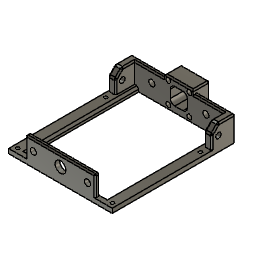
final scissor lift assembly v1 (Autodesk Fusion 360 archive; units mm, degrees)
design "base for scissor lift"
Autodesk Fusion 360 part; units mm, degrees
(part 1 of 2)
sketch "Sketch1" plane through (0, 0, 0) normal (0, 0, 1) x (1, 0, 0)
  line L0 (83.5, 80) -> (-83.5, 80)
  line L1 (-83.5, 80) -> (-83.5, -80)
  line L2 (-83.5, -80) -> (83.5, -80)
  line L3 (83.5, -80) -> (83.5, 80)
  line L4 (83.5, 80) -> (-83.5, -80) construction
  line L5 (-83.5, 80) -> (83.5, -80) construction
  line L6 (-83.5, 80) -> (-86.5, 80)
  line L7 (-86.5, 80) -> (-86.5, -80)
  line L8 (-86.5, -80) -> (-83.5, -80)
  line L9 (-83.5, -80) -> (-83.5, 80)
  line L10 (83.5, 80) -> (86.5, 80)
  line L11 (86.5, 80) -> (86.5, -80)
  line L12 (86.5, -80) -> (83.5, -80)
  line L13 (83.5, -80) -> (83.5, 80)
  dimension "d1" = 167
  dimension "d2" = 160
  dimension "d3" = 3
  dimension "d4" = 160
  dimension "d5" = 3
  dimension "d6" = 160
  constraint horizontal L0
  constraint perpendicular L0 L1
  constraint parallel L0 L2
  constraint parallel L1 L3
  constraint coincident L4 origin
  constraint coincident L5 origin
  constraint horizontal L6
  constraint vertical L7
  constraint horizontal L8
  constraint vertical L9
  constraint horizontal L10
  constraint vertical L11
  constraint horizontal L12
  constraint vertical L13
  measures "d1" distance of L1.end L2.end
  measures "d2" distance of L0.end L1.end
  measures "d3" distance of L0.end L6.end
  measures "d4" distance of L0.end L1.end
  measures "d5" distance of L0.start L10.end
  measures "d6" distance of L0.start L2.end
extrude "Extrude1" add sketch "Sketch1" along normal blind 20 contours L3 L10 L11 L12 L13 | L1 L6 L7 L8 L9 makes body 1 at (86.5, 26.6667, 6.6667) makes body 2 at (-86.5, 26.6667, 6.6667)
sketch "Sketch2" plane through (86.5, 0, 0) normal (1, 0, 0) x (0, 1, 0)
  line L0 (-80, 0) -> (80, 0)
  line L1 (80, 0) -> (80, 20)
  line L2 (80, 20) -> (-80, 20)
  line L3 (-80, 20) -> (-80, 0)
  circle A0 centre (69.9537, 12.5) radius 4
  dimension "d9" = 8
  measures "d9" diameter of A0
extrude "Extrude2" cut sketch "Sketch2" against normal blind 181 contours A0 bodies 1 2
extrude "Extrude4" add sketch "Sketch1" against normal blind 2 bodies 1 2
sketch "Sketch6" plane through (83.5, 0, 0) normal (-1, 0, 0) x (0, -1, 0)
  circle A0 centre (-69.9537, 12.5) radius 4
  line L0 (-80, 0) -> (80, 0)
  line L1 (80, 0) -> (80, 20)
  line L2 (80, 20) -> (-80, 20)
  line L3 (-80, 20) -> (-80, 0)
  line L4 (-80, 20) -> (-60, 20)
  line L5 (-60, 20) -> (-60, 0)
  line L6 (-60, 0) -> (-80, 0)
  line L7 (-80, 0) -> (-80, 20)
  dimension "d31" = 20
  dimension "d32" = 20
  constraint horizontal L4
  constraint vertical L5
  constraint horizontal L6
  constraint vertical L7
  constraint coincident L2.end L3.start
  measures "d31" distance of L2.end L4.end
  measures "d32" distance of L2.end L0.start
extrude "Extrude6" add sketch "Sketch6" along normal blind 18 contours L0 L2 L3 L4 L5 L6 L7 bodies 1
sketch "Sketch7" plane through (-83.5, 0, 0) normal (1, 0, 0) x (0, 1, 0)
  circle A0 centre (69.9537, 12.5) radius 4
  line L0 (-80, 0) -> (80, 0)
  line L1 (80, 0) -> (80, 20)
  line L2 (80, 20) -> (-80, 20)
  line L3 (-80, 20) -> (-80, 0)
  line L4 (80, 20) -> (60, 20)
  line L5 (60, 20) -> (60, 0)
  line L6 (60, 0) -> (80, 0)
  line L7 (80, 0) -> (80, 20)
  dimension "d39" = 20
  dimension "d40" = 20
  constraint horizontal L4
  constraint vertical L5
  constraint horizontal L6
  constraint vertical L7
  constraint coincident L1.end L2.start
  measures "d39" distance of L1.end L4.end
  measures "d40" distance of L1.end L0.end
extrude "Extrude7" add sketch "Sketch7" along normal blind 18 contours L0 L1 L2 L4 L5 L6 L7 bodies 1
sketch "Sketch13" plane through (0, 80, 0) normal (0, 1, 0) x (-1, 0, 0)
  line L0 (-65.5, 20) -> (-86.5, 20)
  line L1 (-86.5, 20) -> (-86.5, -2)
  line L2 (-86.5, -2) -> (86.5, -2)
  line L3 (86.5, -2) -> (86.5, 20)
  line L4 (86.5, 20) -> (65.5, 20)
  line L5 (65.5, 20) -> (65.5, 0)
  line L6 (65.5, 0) -> (-65.5, 0)
  line L7 (-65.5, 0) -> (-65.5, 20)
  line L8 (-86.5, -2) -> (86.5, -2)
  line L9 (86.5, -2) -> (86.5, 20)
  line L10 (86.5, 20) -> (-86.5, 20)
  line L11 (-86.5, 20) -> (-86.5, -2)
  constraint horizontal L8
  constraint vertical L9
  constraint horizontal L10
  constraint vertical L11
  constraint coincident L3.end L4.start
  constraint coincident L1.end L2.start
extrude "Extrude13" add sketch "Sketch13" along normal blind 10 contours L0 L1 L2 L3 L4 L5 L6 L7 L8 L9 L10 L11 bodies 1
extrude "Extrude14" add sketch "Sketch13" along normal blind 2 from surface at 8 contours L5 L6 L7 L10 bodies 1
extrude "Extrude18" cut 1 faces at (-21.8333, -33.3333, 0) along direction (0, 0, -1) blind 2 on bodies 1 bodies 1
sketch "Sketch22" plane through (0, 0, -2) normal (0, 0, -1) x (1, 0, 0)
  line L0 (83.5, 80) -> (83.5, -60)
  line L1 (83.5, -60) -> (65.5, -60)
  line L2 (65.5, -60) -> (65.5, -88)
  line L3 (65.5, -88) -> (-65.5, -88)
  line L4 (-65.5, -88) -> (-65.5, -60)
  line L5 (-65.5, -60) -> (-83.5, -60)
  line L6 (-83.5, -60) -> (-83.5, 80)
  line L7 (-83.5, 80) -> (-86.5, 80)
  line L8 (-86.5, 80) -> (-86.5, -90)
  line L9 (-86.5, -90) -> (86.5, -90)
  line L10 (86.5, -90) -> (86.5, 80)
  line L11 (86.5, 80) -> (83.5, 80)
  line L12 (-86.5, 80) -> (86.5, 80)
  line L13 (86.5, 80) -> (86.5, -90)
  line L14 (86.5, -90) -> (-86.5, -90)
  line L15 (-86.5, -90) -> (-86.5, 80)
  line L16 (86.5, 72.5) -> (103, 72.5)
  line L17 (103, 72.5) -> (103, -82.5)
  line L18 (103, -82.5) -> (86.5, -82.5)
  line L19 (86.5, -82.5) -> (86.5, 72.5)
  line L20 (-86.5, 72.5) -> (-103, 72.5)
  line L21 (-103, 72.5) -> (-103, -82.5)
  line L22 (-103, -82.5) -> (-86.5, -82.5)
  line L23 (-86.5, -82.5) -> (-86.5, 72.5)
  line L24 (-86.5, 80) -> (-91.5, 80)
  line L25 (-91.5, 80) -> (-91.5, 72.5)
  line L26 (-91.5, 72.5) -> (-86.5, 72.5)
  line L27 (-86.5, 72.5) -> (-86.5, 80)
  line L28 (-86.5, -82.5) -> (-91.5, -82.5)
  line L29 (-91.5, -82.5) -> (-91.5, -90)
  line L30 (-91.5, -90) -> (-86.5, -90)
  line L31 (-86.5, -90) -> (-86.5, -82.5)
  line L32 (86.5, 80) -> (91.5, 80)
  line L33 (91.5, 80) -> (91.5, 72.5)
  line L34 (91.5, 72.5) -> (86.5, 72.5)
  line L35 (86.5, 72.5) -> (86.5, 80)
  line L36 (86.5, -90) -> (91.5, -90)
  line L37 (91.5, -90) -> (91.5, -82.5)
  line L38 (91.5, -82.5) -> (86.5, -82.5)
  line L39 (86.5, -82.5) -> (86.5, -90)
  line L40 (-91.5, -90) -> (91.5, -90)
  line L41 (91.5, -90) -> (91.5, -95)
  line L42 (91.5, -95) -> (-91.5, -95)
  line L43 (-91.5, -95) -> (-91.5, -90)
  dimension "d171" = 5
  dimension "d172" = 5
  dimension "d173" = 7.5
  dimension "d174" = 5
  dimension "d175" = 5
  dimension "d176" = 5
  constraint horizontal L12
  constraint vertical L13
  constraint horizontal L14
  constraint vertical L15
  constraint coincident L9.end L10.start
  constraint coincident L7.end L8.start
  constraint horizontal L16
  constraint vertical L17
  constraint horizontal L18
  constraint vertical L19
  constraint coincident L10 L16.start
  constraint horizontal L20
  constraint vertical L21
  constraint horizontal L22
  constraint vertical L23
  constraint coincident L15 L20.start
  constraint horizontal L24
  constraint vertical L25
  constraint horizontal L26
  constraint vertical L27
  constraint horizontal L28
  constraint vertical L29
  constraint horizontal L30
  constraint vertical L31
  constraint horizontal L32
  constraint vertical L33
  constraint horizontal L34
  constraint vertical L35
  constraint horizontal L36
  constraint vertical L37
  constraint horizontal L38
  constraint vertical L39
  constraint horizontal L40
  constraint vertical L41
  constraint horizontal L42
  constraint vertical L43
  measures "d171" distance of L7.end L24.end
  measures "d172" distance of L22.end L28.end
  measures "d173" distance of L28.end L29.end
  measures "d174" distance of L10.end L32.end
  measures "d175" distance of L9.end L36.end
  measures "d176" distance of L29.end L42.end
extrude "Extrude26" add sketch "Sketch22" along normal blind 3 separate body makes body 3
sketch "Sketch23" plane through (0, 0, -2) normal (0, 0, 1) x (-1, 0, 0)
  line L0 (103, 72.5) -> (91.5, 72.5)
  line L1 (91.5, 80) -> (-91.5, 80)
  line L2 (-91.5, 72.5) -> (-103, 72.5)
  line L3 (-103, 72.5) -> (-103, -82.5)
  line L4 (-103, -82.5) -> (-91.5, -82.5)
  line L5 (91.5, -82.5) -> (103, -82.5)
  line L6 (103, -82.5) -> (103, 72.5)
  circle A0 centre (99.32, -80) radius 1.5
  line L7 (91.5, -95) -> (91.5, -82.5)
  line L8 (91.5, 72.5) -> (91.5, 80)
  line L9 (-91.5, 80) -> (-91.5, 72.5)
  line L10 (-91.5, -82.5) -> (-91.5, -95)
  line L11 (-91.5, -95) -> (91.5, -95)
  dimension "d143" = 3
  measures "d143" diameter of A0
extrude "Extrude27" cut sketch "Sketch23" against normal blind 3 contours A0 bodies 3
pattern_linear "R-Pattern5" count 20 spacing 7.8947 along (0, -1, 0) of "Extrude27"
extrude "Extrude29" add 1 faces at (78.5, 79.3333, 20) along direction (0, 0, 1) blind 8 on bodies 1 bodies 1
move_face "OffsetFaces1" offset 5 3 faces at (86.5, -31.3488, 12.8333) (28.8333, 90, 8) (-86.5, -31.3488, 12.8333) on bodies 1
sketch "Sketch30" plane through (0, -80, 0) normal (0, -1, 0) x (1, 0, 0)
  line L0 (-83.5, -2) -> (-83.5, 28)
  line L1 (-83.5, 28) -> (-91.5, 28)
  line L2 (-91.5, 28) -> (-91.5, -2)
  line L3 (-91.5, -2) -> (-83.5, -2)
  line L4 (-91.5, 28) -> (91.5, 28)
  line L5 (91.5, 28) -> (91.5, -2)
  line L6 (91.5, -2) -> (-91.5, -2)
  line L7 (-91.5, -2) -> (-91.5, 28)
  constraint horizontal L4
  constraint vertical L5
  constraint horizontal L6
  constraint vertical L7
  constraint coincident L1.end L2.start
extrude "Extrude36" add sketch "Sketch30" along normal blind 7 bodies 1
sketch "Sketch31" plane through (0, -87, 0) normal (0, -1, 0) x (1, 0, 0)
  line L0 (-91.5, -2) -> (91.5, -2)
  line L1 (91.5, -2) -> (91.5, 28)
  line L2 (91.5, 28) -> (-91.5, 28)
  line L3 (-91.5, 28) -> (-91.5, -2)
  circle A0 centre (0, 12.5) radius 8
  dimension "d193" = 16
  measures "d193" diameter of A0
extrude "Extrude37" cut sketch "Sketch31" against normal blind 7 contours A0 bodies 1
sketch "Sketch32" plane through (0, -87, 0) normal (0, -1, 0) x (1, 0, 0)
  circle A0 centre (0, 12.5) radius 8
  line L0 (-91.5, -2) -> (91.5, -2)
  line L1 (91.5, -2) -> (91.5, 28)
  line L2 (91.5, 28) -> (-91.5, 28)
  line L3 (-91.5, 28) -> (-91.5, -2)
  circle A1 centre (-40, 12.5) radius 4.5
  circle A2 centre (40, 12.5) radius 4.5
  line L4 (40, 12.5) -> (0, 12.5)
  line L5 (0, 12.5) -> (-40, 12.5)
  dimension "d206" = 9
  dimension "d207" = 9
  dimension "d214" = 40
  dimension "d215" = 40
  constraint coincident A2.centre L4.start
  constraint parallel L2 L4
  constraint parallel L4 L5
  measures "d206" diameter of A1
  measures "d207" diameter of A2
  measures "d214" distance of A2.centre A0.centre
  measures "d215" distance of A0.centre A1.centre
extrude "Extrude38" cut sketch "Sketch32" against normal blind 182 contours A1 | A2 bodies 1
sketch "Sketch35" plane through (0, 0, -2) normal (0, 0, -1) x (1, 0, 0)
  line L0 (-91.5, 87) -> (-91.5, -95)
  line L1 (-91.5, -95) -> (91.5, -95)
  line L2 (91.5, -95) -> (91.5, 87)
  line L3 (91.5, 87) -> (-91.5, 87)
  line L4 (-83.5, 80) -> (83.5, 80)
  line L5 (83.5, 80) -> (83.5, -60)
  line L6 (83.5, -60) -> (65.5, -60)
  line L7 (65.5, -60) -> (65.5, -88)
  line L8 (65.5, -88) -> (-65.5, -88)
  line L9 (-65.5, -88) -> (-65.5, -60)
  line L10 (-65.5, -60) -> (-83.5, -60)
  line L11 (-83.5, -60) -> (-83.5, 80)
  line L12 (-91.5, 87) -> (91.5, 87)
  line L13 (91.5, 87) -> (91.5, -95)
  line L14 (91.5, -95) -> (-91.5, -95)
  line L15 (-91.5, -95) -> (-91.5, 87)
  line L16 (-49.9161, -98) -> (-91.5, -98)
  line L17 (-91.5, -98) -> (-91.5, -95)
  line L18 (-91.5, -95) -> (-49.9161, -95)
  line L19 (-49.9161, -95) -> (-49.9161, -98)
  constraint horizontal L12
  constraint vertical L13
  constraint horizontal L14
  constraint vertical L15
  constraint coincident L1.end L2.start
  constraint coincident L0.start L3.end
  constraint horizontal L16
  constraint vertical L17
  constraint horizontal L18
  constraint vertical L19
  constraint coincident L0.end L1.start
extrude "Extrude41" add sketch "Sketch35" along normal blind 6.65 contours L0 L1 L2 L3 L12 L13 L14 L15 L18 | L4 L5 L6 L7 L8 L9 L10 L11 bodies 1
sketch "Sketch36" plane through (0, 0, -2) normal (0, 0, 1) x (-1, 0, 0)
  line L0 (65.5, -60) -> (83.5, -60)
  line L1 (83.5, -60) -> (83.5, 80)
  line L2 (83.5, 80) -> (-83.5, 80)
  line L3 (-83.5, 80) -> (-83.5, -60)
  line L4 (-83.5, -60) -> (-65.5, -60)
  line L5 (-65.5, -60) -> (-65.5, -88)
  line L6 (-65.5, -88) -> (65.5, -88)
  line L7 (65.5, -88) -> (65.5, -60)
sketch "Sketch37" plane through (0, 0, -2) normal (0, 0, 1) x (-1, 0, 0)
  line L0 (65.5, -60) -> (83.5, -60)
  line L1 (83.5, -60) -> (83.5, 80)
  line L2 (83.5, 80) -> (-83.5, 80)
  line L3 (-83.5, 80) -> (-83.5, -60)
  line L4 (-83.5, -60) -> (-65.5, -60)
  line L5 (-65.5, -60) -> (-65.5, -88)
  line L6 (-65.5, -88) -> (65.5, -88)
  line L7 (65.5, -88) -> (65.5, -60)
  line L8 (-83.5, 80) -> (-59.3, 80)
  line L9 (-59.3, 80) -> (-59.3, -88)
  line L10 (-59.3, -88) -> (-83.5, -88)
  line L11 (-83.5, -88) -> (-83.5, 80)
  line L12 (83.5, 80) -> (59.3, 80)
  line L13 (59.3, 80) -> (59.3, -88)
  line L14 (59.3, -88) -> (83.5, -88)
  line L15 (83.5, -88) -> (83.5, 80)
  dimension "d264" = 24.2
  dimension "d265" = 24.2
  dimension "d266" = 168
  dimension "d267" = 168
  constraint horizontal L8
  constraint vertical L9
  constraint horizontal L10
  constraint vertical L11
  constraint coincident L6 L9.end
  constraint coincident L2.end L3.start
  constraint horizontal L12
  constraint vertical L13
  constraint horizontal L14
  constraint vertical L15
  constraint coincident L1.end L2.start
  measures "d264" distance of L2.end L8.end
  measures "d265" distance of L1.end L12.end
  measures "d266" distance of L8.end L9.end
  measures "d267" distance of L12.end L13.end
extrude "Extrude43" cut sketch "Sketch37" against normal blind 6.65 contours L2 L6 L9 L13 bodies 1
chamfer "Chamfer2" distance 3 angle 45 2 edges at (-59.3, 4, -2) (59.3, 4, -2) on bodies 1
sketch "Sketch39" plane through (0, 95, 0) normal (0, 1, 0) x (-1, 0, 0)
  circle A0 centre (-31.5, 2.5) radius 1.4
  circle A1 centre (31.5, 12.5) radius 1.4
  circle A2 centre (0, 22.5) radius 1.4
  circle A3 centre (-31.5, 12.5) radius 1.4
  circle A4 centre (0, 2.5) radius 1.4
  circle A5 centre (31.5, 22.5) radius 1.4
  circle A6 centre (31.5, 2.5) radius 1.4
  circle A7 centre (-31.5, 22.5) radius 1.4
  circle A8 centre (0, 12.5) radius 4.5
  circle A9 centre (-40, 12.5) radius 4.5
  circle A10 centre (40, 12.5) radius 4.5
  line L0 (-91.5, 28) -> (-91.5, -8.65)
  line L1 (-91.5, -8.65) -> (91.5, -8.65)
  line L2 (91.5, -8.65) -> (91.5, 28)
  line L3 (91.5, 28) -> (-91.5, 28)
  line L4 (-21.15, 33.65) -> (21.15, 33.65)
  line L5 (21.15, 33.65) -> (21.15, -8.65)
  line L6 (21.15, -8.65) -> (-21.15, -8.65)
  line L7 (-21.15, -8.65) -> (-21.15, 33.65)
  circle A11 centre (15.5, 28) radius 1.6
  circle A12 centre (-15.5, 28) radius 1.6
  circle A13 centre (15.5, -3) radius 1.6
  circle A14 centre (-15.5, -3) radius 1.6
  circle A15 centre (-40, 12.5) radius 4.5
  circle A16 centre (40, 12.5) radius 4.5
  circle A17 centre (0, 12.5) radius 8
  line L8 (83.5, -2) -> (83.5, 28)
  line L9 (83.5, 28) -> (-83.5, 28)
  line L10 (-83.5, 28) -> (-83.5, -2)
  line L11 (-83.5, -2) -> (-62.3, -2)
  line L12 (-62.3, -2) -> (-59.3, -5)
  line L13 (-59.3, -5) -> (-59.3, -8.65)
  line L14 (-59.3, -8.65) -> (59.3, -8.65)
  line L15 (59.3, -8.65) -> (59.3, -5)
  line L16 (59.3, -5) -> (62.3, -2)
  line L17 (62.3, -2) -> (83.5, -2)
  circle A18 centre (-40, 12.5) radius 4.5
  circle A19 centre (40, 12.5) radius 4.5
  line L18 (-91.5, 28) -> (-91.5, -8.65)
  line L19 (-91.5, -8.65) -> (91.5, -8.65)
  line L20 (91.5, -8.65) -> (91.5, 28)
  line L21 (91.5, 28) -> (-91.5, 28)
  point P0 (0, 12.5)
  dimension "d287" = 42.3
  dimension "d288" = 3.2
  dimension "d289" = 3.2
  dimension "d290" = 3.2
  dimension "d291" = 3.2
  constraint horizontal L4
  constraint perpendicular L4 L5
  constraint parallel L4 L6
  constraint parallel L5 L7
  constraint coincident P0 A8.centre
  constraint coincident L3 A11.centre
  constraint coincident L3 A12.centre
  measures "d287" distance of L5.end L6.end
  measures "d288" diameter of A11
  measures "d289" diameter of A12
  measures "d290" diameter of A13
  measures "d291" diameter of A14
extrude "Extrude45" add sketch "Sketch39" against normal blind 7 contours L3 L4 L5 L7 A11 A12 L9 L21 bodies 1
extrude "Extrude46" cut sketch "Sketch39" against normal blind 7 contours L3 A12 L9 L21 | L3 A11 L9 L21 | A13 | A14 picked at (-15.6948, 27.5035) picked at (15.3052, 27.3446) bodies 1
extrude "Extrude48" cut 1 faces at (-83.5, 13.3333, 8) along direction (1, 0, 0) blind -30 and the other way blind -220 on bodies 1 bodies 1
sketch "Sketch41" plane through (0, 95, 0) normal (0, -1, 0) x (1, 0, 0)
  circle A0 centre (40, 12.5) radius 4.5
  circle A1 centre (-40, 12.5) radius 4.5
  line L0 (21.15, 28) -> (21.15, 33.65)
  line L1 (21.15, 33.65) -> (-21.15, 33.65)
  line L2 (-21.15, 33.65) -> (-21.15, 28)
  line L3 (-21.15, 28) -> (-65.5, 28)
  line L4 (-59.3, -8.65) -> (59.3, -8.65)
  line L5 (65.5, 28) -> (21.15, 28)
  line L6 (-21.15, 33.65) -> (21.15, 33.65)
  line L7 (21.15, 33.65) -> (21.15, -8.65)
  line L8 (21.15, -8.65) -> (-21.15, -8.65)
  line L9 (-21.15, -8.65) -> (-21.15, 33.65)
  line L10 (-21.15, 33.65) -> (21.15, -8.65) construction
  line L11 (21.15, 33.65) -> (-21.15, -8.65) construction
  line L12 (-12.5, 25) -> (12.5, 25)
  line L13 (12.5, 25) -> (12.5, 0)
  line L14 (12.5, 0) -> (-12.5, 0)
  line L15 (-12.5, 0) -> (-12.5, 25)
  line L16 (-12.5, 25) -> (12.5, 0) construction
  line L17 (12.5, 25) -> (-12.5, 0) construction
  circle A2 centre (0, 12.5) radius 4.5
  line L18 (-65.5, 28) -> (-65.5, -2)
  line L19 (-65.5, -2) -> (-62.3, -2)
  line L20 (-62.3, -2) -> (-59.3, -5)
  line L21 (-59.3, -5) -> (-59.3, -8.65)
  line L22 (59.3, -8.65) -> (59.3, -5)
  line L23 (59.3, -5) -> (62.3, -2)
  line L24 (62.3, -2) -> (65.5, -2)
  line L25 (65.5, -2) -> (65.5, 28)
  circle A3 centre (15.5, 28) radius 1.6
  circle A4 centre (-15.5, 28) radius 1.6
  circle A5 centre (15.5, -3) radius 1.6
  circle A6 centre (-15.5, -3) radius 1.6
  line L26 (21.15, 28) -> (91.5, 28)
  line L27 (91.5, 28) -> (91.5, -8.65)
  line L28 (91.5, -8.65) -> (-91.5, -8.65)
  line L29 (-91.5, -8.65) -> (-91.5, 28)
  line L30 (-91.5, 28) -> (-21.15, 28)
  line L31 (-21.15, 28) -> (-21.15, 33.65)
  line L32 (-21.15, 33.65) -> (21.15, 33.65)
  line L33 (21.15, 33.65) -> (21.15, 28)
  circle A7 centre (40, 12.5) radius 4.5
  circle A8 centre (-40, 12.5) radius 4.5
  point P0 (0, 12.5)
  point P1 (0, 12.5)
  dimension "d308" = 25
  dimension "d309" = 25
  constraint horizontal L6
  constraint perpendicular L6 L7
  constraint parallel L6 L8
  constraint parallel L7 L9
  constraint coincident L10 P1
  constraint coincident L11 P1
  constraint coincident L1.end L2.start
  constraint horizontal L12
  constraint perpendicular L12 L13
  constraint parallel L12 L14
  constraint parallel L13 L15
  constraint coincident L16 P1
  constraint coincident L17 P1
  measures "d308" distance of L13.end L14.end
  measures "d309" distance of L12.end L13.end
extrude "Extrude49" add sketch "Sketch41" against normal blind 17.7 contours L0 L1 L2 L4 L6 L7 L8 L9 L28 L31 L32 L33 bodies 1
sketch "Sketch42" plane through (0, -80, 0) normal (0, 1, 0) x (-1, 0, 0)
  line L0 (91.5, 28) -> (-91.5, 28)
  line L1 (-91.5, 28) -> (-91.5, -2)
  line L2 (-91.5, -2) -> (-62.3, -2)
  line L3 (-62.3, -2) -> (-59.3, -5)
  line L4 (-59.3, -5) -> (-59.3, -8.65)
  line L5 (-59.3, -8.65) -> (59.3, -8.65)
  line L6 (59.3, -8.65) -> (59.3, -5)
  line L7 (59.3, -5) -> (62.3, -2)
  line L8 (62.3, -2) -> (91.5, -2)
  line L9 (91.5, -2) -> (91.5, 28)
  circle A0 centre (0, 12.5) radius 8
  circle A1 centre (40, 12.5) radius 4.5
  circle A2 centre (-40, 12.5) radius 4.5
  line L10 (-91.5, 28) -> (-51.5, 28)
  line L11 (-51.5, 28) -> (-51.5, -2)
  line L12 (-51.5, -2) -> (-91.5, -2)
  line L13 (-91.5, -2) -> (-91.5, 28)
  line L14 (91.5, 28) -> (51.5, 28)
  line L15 (51.5, 28) -> (51.5, -2)
  line L16 (51.5, -2) -> (91.5, -2)
  line L17 (91.5, -2) -> (91.5, 28)
  dimension "d312" = 40
  dimension "d313" = 40
  constraint horizontal L10
  constraint vertical L11
  constraint horizontal L12
  constraint vertical L13
  constraint coincident L0.end L1.start
  constraint horizontal L14
  constraint vertical L15
  constraint horizontal L16
  constraint vertical L17
  constraint coincident L0.start L9.end
  measures "d312" distance of L0.end L10.end
  measures "d313" distance of L0.start L14.end
extrude "Extrude50" cut sketch "Sketch42" against normal blind 35 contours L0 L8 L9 L14 L15 L16 L17 | L0 L1 L2 L10 L11 L12 L13 bodies 1
extrude "Extrude51" cut 2 faces at (91.5, 22.6667, -6.4333) (91.5, 87.9846, 12.8333) along direction (-1, 0, 0) blind 15 on bodies 1 bodies 1
extrude "Extrude52" cut 1 faces at (-91.5, 87.9697, 10.4179) along direction (1, 0, 0) blind 15 on bodies 1 bodies 1
chamfer "Chamfer3" distance 10 angle 45 2 edges at (-71, 60, 28) (71, 60, 28) on bodies 1
chamfer "Chamfer4" distance 2 angle 45 41 edges at (-65.5, 60, 8) (-76.5, 60, 8) (-76.5, 65, 23) (-71, 60, 18) (-65.5, 65, 23) (-71, 70, 28) (-76.5, 82.5, 28) (-65.5, 79, 28) (-48.825, 95, 28) (48.825, 95, 28) (43.325, 88, 28) (-43.325, 88, 28) (76.5, 82.5, 28) (65.5, 79, 28) (65.5, 65, 23) (71, 70, 28) (76.5, 65, 23) (71, 60, 18) (65.5, 60, 8) (76.5, 60, 8) (76.5, 95, 9.675) (-76.5, 95, 9.675) (56.325, 95, 28) (0, -80, 28) (43.325, 88, 28) (0, -87, 28) (51.5, -83.5, 28) (-43.325, 88, 28) (0, -87, 28) (-51.5, -83.5, 28) (-56.325, 95, 28) (0, -80, 28) (51.5, -87, 13) (51.5, -80, 13) (-51.5, -80, 13) (-51.5, -87, 13) (-21.15, 112.7, 12.5) (21.15, 112.7, 12.5) (-21.15, 103.85, -8.65) (21.15, 103.85, -8.65) (0, 112.7, -8.65) 1 faces at (-7.05, 96.2333, 33.65) on bodies 1
sketch "Sketch44" plane through (0, 0, -2) normal (0, 0, 1) x (-1, 0, 0)
  line L0 (76.5, -62) -> (76.5, 87)
  line L1 (76.5, 87) -> (49.5, 87)
  line L2 (49.5, 87) -> (51.5, 85)
  line L3 (51.5, 85) -> (51.5, 82)
  line L4 (51.5, 82) -> (49.5, 80)
  line L5 (49.5, 80) -> (62.3, 80)
  line L6 (62.3, 80) -> (62.3, -88)
  line L7 (62.3, -88) -> (65.5, -88)
  line L8 (65.5, -88) -> (65.5, -62)
  line L9 (65.5, -62) -> (67.5, -60)
  line L10 (67.5, -60) -> (74.5, -60)
  line L11 (74.5, -60) -> (76.5, -62)
  circle A0 centre (-70, 80) radius 2.5
  dimension "d322" = 5
  measures "d322" diameter of A0
extrude "Extrude53" cut sketch "Sketch44" against normal blind 10 contours A0 bodies 1
pattern_linear "R-Pattern7" count 2 spacing 130 along (0, 1, 0) count 2 spacing 140 along (-1, 0, 0) of "Extrude53"
sketch "Sketch45" plane through (0, 88, 0) normal (0, -1, 0) x (1, 0, 0)
  line L0 (21.15, 31.65) -> (-21.15, 31.65)
  line L1 (-21.15, 31.65) -> (-21.15, 26)
  line L2 (-21.15, 26) -> (-65.5, 26)
  line L3 (-65.5, 26) -> (-65.5, -2)
  line L4 (-65.5, -2) -> (-62.3, -2)
  line L5 (-62.3, -2) -> (-59.3, -5)
  line L6 (-59.3, -5) -> (-59.3, -8.65)
  line L7 (-59.3, -8.65) -> (59.3, -8.65)
  line L8 (59.3, -8.65) -> (59.3, -5)
  line L9 (59.3, -5) -> (62.3, -2)
  line L10 (62.3, -2) -> (65.5, -2)
  line L11 (65.5, -2) -> (65.5, 26)
  line L12 (65.5, 26) -> (21.15, 26)
  line L13 (21.15, 26) -> (21.15, 31.65)
  circle A0 centre (15.5, -3) radius 1.6
  circle A1 centre (-15.5, -3) radius 1.6
  circle A2 centre (15.5, 28) radius 1.6
  circle A3 centre (-15.5, 28) radius 1.6
  circle A4 centre (40, 12.5) radius 4.5
  circle A5 centre (-40, 12.5) radius 4.5
  circle A6 centre (-15.5, 28) radius 3.5
  circle A7 centre (-15.5, -3) radius 3.5
  circle A8 centre (15.5, -3) radius 3.5
  circle A9 centre (15.5, 28) radius 3.5
  dimension "d329" = 7
  dimension "d330" = 7
  dimension "d331" = 7
  dimension "d332" = 7
  constraint concentric A3 A6
  constraint concentric A1 A7
  constraint concentric A0 A8
  constraint concentric A2 A9
  measures "d329" diameter of A6
  measures "d330" diameter of A7
  measures "d331" diameter of A8
  measures "d332" diameter of A9
extrude "Extrude54" cut sketch "Sketch45" against normal blind 15.7 contours A6 | A7 | A8 | A9 bodies 1
extrude "Extrude55" cut 1 faces at (-4.1667, 95, 8.3333) along direction (0, -1, 0) blind 7 on bodies 1 bodies 1
fillet "Fillet2" radius 6.5 4 edges at (-12.5, 100.35, 25) (-12.5, 100.35, 0) (12.5, 100.35, 25) (12.5, 100.35, 0) on bodies 1
sketch "Sketch46" plane through (0, 0, 0) normal (0, 0, 1) x (1, 0, 0)
  line L0 (-21, 88) -> (-21, 113)
  line L1 (-21, 113) -> (-80, 113)
  line L2 (-80, 113) -> (-80, -100)
  line L3 (-80, -100) -> (100, -100)
  line L4 (100, -100) -> (100, 100)
  line L5 (100, 100) -> (21.9148, 113)
  line L6 (21.9148, 113) -> (21.9148, 88.2807)
  line L7 (21.9148, 88.2807) -> (-21, 88)
  constraint vertical L0
  constraint perpendicular L0 L1
  constraint perpendicular L1 L2
  constraint perpendicular L2 L3
  constraint perpendicular L3 L4
  constraint parallel L4 L6
sketch "Sketch47" plane through (0, 95, 0) normal (0, 1, 0) x (-1, 0, 0)
  line L0 (-74.5, 26) -> (-74.5, -8.65)
  line L1 (-74.5, -8.65) -> (-19.15, -8.65)
  line L2 (-19.15, -8.65) -> (-21.15, -6.65)
  line L3 (-21.15, -6.65) -> (-21.15, 26)
  line L4 (-21.15, 26) -> (-74.5, 26)
  circle A0 centre (-40, 12.5) radius 4.5
  circle A1 centre (-40, 12.5) radius 6
  circle A2 centre (40, 12.5) radius 6
  dimension "d343" = 12
  dimension "d344" = 12
  constraint concentric A0 A1
  measures "d343" diameter of A1
  measures "d344" diameter of A2
extrude "Extrude58" add sketch "Sketch47" along normal blind 2 contours A0 | A1 | A2 bodies 1
fillet "Fillet3" radius 2 2 edges at (-34.406, 95, 14.6697) (45.594, 95, 14.6697) on bodies 1
hidden bodies 3
equation "d264 = 12.100 * 2 mm"
equation "d333 = -20.00 mm + 4.3 mm"

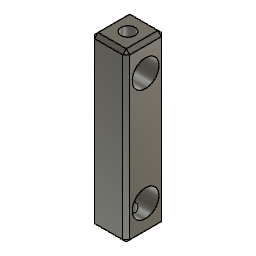
design "small slider"
Autodesk Fusion 360 part; units mm, degrees
sketch "Sketch1" plane through (0, 0, 0) normal (0, 0, 1) x (1, 0, 0)
  line L0 (10, -11) -> (-10, -11)
  line L1 (-10, -11) -> (-10, 11)
  line L2 (-10, 11) -> (10, 11)
  line L3 (10, 11) -> (10, -11)
  line L4 (10, -11) -> (-10, 11) construction
  line L5 (-10, -11) -> (10, 11) construction
  circle A0 centre (0, 0) radius 4
  dimension "d1" = 20
  dimension "d2" = 22
  dimension "d75" = 8
  constraint horizontal L0
  constraint perpendicular L0 L1
  constraint parallel L0 L2
  constraint parallel L1 L3
  measures "d1" distance of L1.end L2.end
  measures "d2" distance of L0.end L1.end
  measures "d75" diameter of A0
extrude "Extrude1" add sketch "Sketch1" along normal blind 95 contours L0 L1 L2 L3 | A0
sketch "Sketch3" plane through (0, 0, 95) normal (0, 0, 1) x (-1, 0, 0)
  line L0 (-10, -11) -> (10, -11)
  line L1 (10, -11) -> (10, 11)
  line L2 (10, 11) -> (-10, 11)
  line L3 (-10, 11) -> (-10, -11)
  circle A0 centre (0, 0) radius 4
  dimension "d21" = 8
  measures "d21" diameter of A0
extrude "Extrude5" cut sketch "Sketch3" against normal blind 10 contours A0
extrude "Extrude6" cut sketch "Sketch1" along normal blind 10 contours A0
sketch "Sketch5" plane through (10, 0, 0) normal (1, 0, 0) x (0, 1, 0)
  line L0 (-11, 0) -> (11, 0)
  line L1 (11, 0) -> (11, 95)
  line L2 (-11, 95) -> (-11, 0)
  circle A0 centre (0, 15.5) radius 7.6
  circle A1 centre (0, 79.5) radius 7.6
  line L3 (11, 95) -> (-11, 95)
  line L4 (0, 95) -> (0, 79.5)
  dimension "d41" = 15.2
  dimension "d43" = 15.2
  dimension "d97" = 15.5
  constraint midpoint L3 L4.start
  constraint perpendicular L3 L4
  measures "d41" diameter of A0
  measures "d43" diameter of A1
  measures "d97" distance of L4.start A1.centre
extrude "Extrude8" cut sketch "Sketch5" against normal blind 20 contours A0 | A1
sketch "Sketch6" plane through (-10, 0, 0) normal (-1, 0, 0) x (0, -1, 0)
  circle A0 centre (0, 15.5) radius 7.6
  line L0 (-11, 0) -> (11, 0)
  line L1 (11, 0) -> (11, 95)
  line L2 (-11, 95) -> (-11, 0)
  circle A1 centre (0, 15.5) radius 9
  circle A2 centre (0, 79.5) radius 9
  circle A3 centre (0, 79.5) radius 4.2
  circle A4 centre (0, 15.5) radius 4.2
  line L3 (11, 95) -> (-11, 95)
  circle A5 centre (0, 79.5) radius 7.6
  dimension "d48" = 18
  dimension "d49" = 18
  dimension "d54" = 8.4
  dimension "d55" = 8.4
  constraint concentric A0 A1
  constraint concentric A2 A3
  constraint concentric A0 A4
  measures "d48" diameter of A1
  measures "d49" diameter of A2
  measures "d54" diameter of A3
  measures "d55" diameter of A4
extrude "Extrude10" add sketch "Sketch6" against normal blind 2 contours A0 | A1 | A2 | A5
chamfer "Chamfer1" distance 2 angle 45 8 edges at (0, 11, 0) (10, 0, 0) (-10, 0, 0) (0, -11, 0) (-10, 0, 95) (0, -11, 95) (10, 0, 95) (0, 11, 95) 2 faces at (3.3333, -11, 31.6667) (-3.3333, 11, 31.6667)

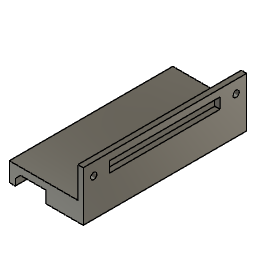
design "slider connector"
Autodesk Fusion 360 part; units mm, degrees
sketch "Sketch1" plane through (0, 0, 0) normal (0, 0, 1) x (1, 0, 0)
  line L0 (83.5, 80) -> (-83.5, 80)
  line L1 (-83.5, 80) -> (-83.5, -80)
  line L2 (-83.5, -80) -> (83.5, -80)
  line L3 (83.5, -80) -> (83.5, 80)
  line L4 (83.5, 80) -> (-83.5, -80) construction
  line L5 (-83.5, 80) -> (83.5, -80) construction
  line L6 (-83.5, 80) -> (-86.5, 80)
  line L7 (-86.5, 80) -> (-86.5, -80)
  line L8 (-86.5, -80) -> (-83.5, -80)
  line L9 (-83.5, -80) -> (-83.5, 80)
  line L10 (83.5, 80) -> (86.5, 80)
  line L11 (86.5, 80) -> (86.5, -80)
  line L12 (86.5, -80) -> (83.5, -80)
  line L13 (83.5, -80) -> (83.5, 80)
  dimension "d1" = 167
  dimension "d2" = 160
  dimension "d3" = 3
  dimension "d4" = 160
  dimension "d5" = 3
  dimension "d6" = 160
  constraint horizontal L0
  constraint perpendicular L0 L1
  constraint parallel L0 L2
  constraint parallel L1 L3
  constraint coincident L4 origin
  constraint coincident L5 origin
  constraint horizontal L6
  constraint vertical L7
  constraint horizontal L8
  constraint vertical L9
  constraint horizontal L10
  constraint vertical L11
  constraint horizontal L12
  constraint vertical L13
  measures "d1" distance of L1.end L2.end
  measures "d2" distance of L0.end L1.end
  measures "d3" distance of L0.end L6.end
  measures "d4" distance of L0.end L1.end
  measures "d5" distance of L0.start L10.end
  measures "d6" distance of L0.start L2.end
extrude "Extrude1" add sketch "Sketch1" along normal blind 20 contours L3 L10 L11 L12 L13 | L1 L6 L7 L8 L9 makes body 1 at (86.5, 26.6667, 6.6667) makes body 2 at (-86.5, 26.6667, 6.6667)
sketch "Sketch2" plane through (86.5, 0, 0) normal (1, 0, 0) x (0, 1, 0)
  line L0 (-80, 0) -> (80, 0)
  line L1 (80, 0) -> (80, 20)
  line L2 (80, 20) -> (-80, 20)
  line L3 (-80, 20) -> (-80, 0)
  circle A0 centre (69.9537, 12.5) radius 4
  dimension "d9" = 8
  measures "d9" diameter of A0
extrude "Extrude2" cut sketch "Sketch2" against normal blind 181 contours A0 bodies 1 2
extrude "Extrude4" add sketch "Sketch1" against normal blind 2 bodies 1 2
sketch "Sketch6" plane through (83.5, 0, 0) normal (-1, 0, 0) x (0, -1, 0)
  circle A0 centre (-69.9537, 12.5) radius 4
  line L0 (-80, 0) -> (80, 0)
  line L1 (80, 0) -> (80, 20)
  line L2 (80, 20) -> (-80, 20)
  line L3 (-80, 20) -> (-80, 0)
  line L4 (-80, 20) -> (-60, 20)
  line L5 (-60, 20) -> (-60, 0)
  line L6 (-60, 0) -> (-80, 0)
  line L7 (-80, 0) -> (-80, 20)
  dimension "d31" = 20
  dimension "d32" = 20
  constraint horizontal L4
  constraint vertical L5
  constraint horizontal L6
  constraint vertical L7
  constraint coincident L2.end L3.start
  measures "d31" distance of L2.end L4.end
  measures "d32" distance of L2.end L0.start
extrude "Extrude6" add sketch "Sketch6" along normal blind 18 contours L0 L2 L3 L4 L5 L6 L7 bodies 1
sketch "Sketch7" plane through (-83.5, 0, 0) normal (1, 0, 0) x (0, 1, 0)
  circle A0 centre (69.9537, 12.5) radius 4
  line L0 (-80, 0) -> (80, 0)
  line L1 (80, 0) -> (80, 20)
  line L2 (80, 20) -> (-80, 20)
  line L3 (-80, 20) -> (-80, 0)
  line L4 (80, 20) -> (60, 20)
  line L5 (60, 20) -> (60, 0)
  line L6 (60, 0) -> (80, 0)
  line L7 (80, 0) -> (80, 20)
  dimension "d39" = 20
  dimension "d40" = 20
  constraint horizontal L4
  constraint vertical L5
  constraint horizontal L6
  constraint vertical L7
  constraint coincident L1.end L2.start
  measures "d39" distance of L1.end L4.end
  measures "d40" distance of L1.end L0.end
extrude "Extrude7" add sketch "Sketch7" along normal blind 18 contours L0 L1 L2 L4 L5 L6 L7 bodies 1
sketch "Sketch13" plane through (0, 80, 0) normal (0, 1, 0) x (-1, 0, 0)
  line L0 (-65.5, 20) -> (-86.5, 20)
  line L1 (-86.5, 20) -> (-86.5, -2)
  line L2 (-86.5, -2) -> (86.5, -2)
  line L3 (86.5, -2) -> (86.5, 20)
  line L4 (86.5, 20) -> (65.5, 20)
  line L5 (65.5, 20) -> (65.5, 0)
  line L6 (65.5, 0) -> (-65.5, 0)
  line L7 (-65.5, 0) -> (-65.5, 20)
  line L8 (-86.5, -2) -> (86.5, -2)
  line L9 (86.5, -2) -> (86.5, 20)
  line L10 (86.5, 20) -> (-86.5, 20)
  line L11 (-86.5, 20) -> (-86.5, -2)
  constraint horizontal L8
  constraint vertical L9
  constraint horizontal L10
  constraint vertical L11
  constraint coincident L3.end L4.start
  constraint coincident L1.end L2.start
extrude "Extrude13" add sketch "Sketch13" along normal blind 10 contours L0 L1 L2 L3 L4 L5 L6 L7 L8 L9 L10 L11 bodies 1
extrude "Extrude14" add sketch "Sketch13" along normal blind 2 from surface at 8 contours L5 L6 L7 L10 bodies 1
extrude "Extrude18" cut 1 faces at (-21.8333, -33.3333, 0) along direction (0, 0, -1) blind 2 on bodies 1 bodies 1
sketch "Sketch22" plane through (0, 0, -2) normal (0, 0, -1) x (1, 0, 0)
  line L0 (83.5, 80) -> (83.5, -60)
  line L1 (83.5, -60) -> (65.5, -60)
  line L2 (65.5, -60) -> (65.5, -88)
  line L3 (65.5, -88) -> (-65.5, -88)
  line L4 (-65.5, -88) -> (-65.5, -60)
  line L5 (-65.5, -60) -> (-83.5, -60)
  line L6 (-83.5, -60) -> (-83.5, 80)
  line L7 (-83.5, 80) -> (-86.5, 80)
  line L8 (-86.5, 80) -> (-86.5, -90)
  line L9 (-86.5, -90) -> (86.5, -90)
  line L10 (86.5, -90) -> (86.5, 80)
  line L11 (86.5, 80) -> (83.5, 80)
  line L12 (-86.5, 80) -> (86.5, 80)
  line L13 (86.5, 80) -> (86.5, -90)
  line L14 (86.5, -90) -> (-86.5, -90)
  line L15 (-86.5, -90) -> (-86.5, 80)
  line L16 (86.5, 72.5) -> (103, 72.5)
  line L17 (103, 72.5) -> (103, -82.5)
  line L18 (103, -82.5) -> (86.5, -82.5)
  line L19 (86.5, -82.5) -> (86.5, 72.5)
  line L20 (-86.5, 72.5) -> (-103, 72.5)
  line L21 (-103, 72.5) -> (-103, -82.5)
  line L22 (-103, -82.5) -> (-86.5, -82.5)
  line L23 (-86.5, -82.5) -> (-86.5, 72.5)
  line L24 (-86.5, 80) -> (-91.5, 80)
  line L25 (-91.5, 80) -> (-91.5, 72.5)
  line L26 (-91.5, 72.5) -> (-86.5, 72.5)
  line L27 (-86.5, 72.5) -> (-86.5, 80)
  line L28 (-86.5, -82.5) -> (-91.5, -82.5)
  line L29 (-91.5, -82.5) -> (-91.5, -90)
  line L30 (-91.5, -90) -> (-86.5, -90)
  line L31 (-86.5, -90) -> (-86.5, -82.5)
  line L32 (86.5, 80) -> (91.5, 80)
  line L33 (91.5, 80) -> (91.5, 72.5)
  line L34 (91.5, 72.5) -> (86.5, 72.5)
  line L35 (86.5, 72.5) -> (86.5, 80)
  line L36 (86.5, -90) -> (91.5, -90)
  line L37 (91.5, -90) -> (91.5, -82.5)
  line L38 (91.5, -82.5) -> (86.5, -82.5)
  line L39 (86.5, -82.5) -> (86.5, -90)
  line L40 (-91.5, -90) -> (91.5, -90)
  line L41 (91.5, -90) -> (91.5, -95)
  line L42 (91.5, -95) -> (-91.5, -95)
  line L43 (-91.5, -95) -> (-91.5, -90)
  dimension "d171" = 5
  dimension "d172" = 5
  dimension "d173" = 7.5
  dimension "d174" = 5
  dimension "d175" = 5
  dimension "d176" = 5
  constraint horizontal L12
  constraint vertical L13
  constraint horizontal L14
  constraint vertical L15
  constraint coincident L9.end L10.start
  constraint coincident L7.end L8.start
  constraint horizontal L16
  constraint vertical L17
  constraint horizontal L18
  constraint vertical L19
  constraint coincident L10 L16.start
  constraint horizontal L20
  constraint vertical L21
  constraint horizontal L22
  constraint vertical L23
  constraint coincident L15 L20.start
  constraint horizontal L24
  constraint vertical L25
  constraint horizontal L26
  constraint vertical L27
  constraint horizontal L28
  constraint vertical L29
  constraint horizontal L30
  constraint vertical L31
  constraint horizontal L32
  constraint vertical L33
  constraint horizontal L34
  constraint vertical L35
  constraint horizontal L36
  constraint vertical L37
  constraint horizontal L38
  constraint vertical L39
  constraint horizontal L40
  constraint vertical L41
  constraint horizontal L42
  constraint vertical L43
  measures "d171" distance of L7.end L24.end
  measures "d172" distance of L22.end L28.end
  measures "d173" distance of L28.end L29.end
  measures "d174" distance of L10.end L32.end
  measures "d175" distance of L9.end L36.end
  measures "d176" distance of L29.end L42.end
extrude "Extrude26" add sketch "Sketch22" along normal blind 3 separate body makes body 3
sketch "Sketch23" plane through (0, 0, -2) normal (0, 0, 1) x (-1, 0, 0)
  line L0 (103, 72.5) -> (91.5, 72.5)
  line L1 (91.5, 80) -> (-91.5, 80)
  line L2 (-91.5, 72.5) -> (-103, 72.5)
  line L3 (-103, 72.5) -> (-103, -82.5)
  line L4 (-103, -82.5) -> (-91.5, -82.5)
  line L5 (91.5, -82.5) -> (103, -82.5)
  line L6 (103, -82.5) -> (103, 72.5)
  circle A0 centre (99.32, -80) radius 1.5
  line L7 (91.5, -95) -> (91.5, -82.5)
  line L8 (91.5, 72.5) -> (91.5, 80)
  line L9 (-91.5, 80) -> (-91.5, 72.5)
  line L10 (-91.5, -82.5) -> (-91.5, -95)
  line L11 (-91.5, -95) -> (91.5, -95)
  dimension "d143" = 3
  measures "d143" diameter of A0
extrude "Extrude27" cut sketch "Sketch23" against normal blind 3 contours A0 bodies 3
pattern_linear "R-Pattern5" count 20 spacing 7.8947 along (0, -1, 0) of "Extrude27"
extrude "Extrude29" add 1 faces at (78.5, 79.3333, 20) along direction (0, 0, 1) blind 8 on bodies 1 bodies 1
move_face "OffsetFaces1" offset 5 3 faces at (86.5, -31.3488, 12.8333) (28.8333, 90, 8) (-86.5, -31.3488, 12.8333) on bodies 1
sketch "Sketch30" plane through (0, -80, 0) normal (0, -1, 0) x (1, 0, 0)
  line L0 (-83.5, -2) -> (-83.5, 28)
  line L1 (-83.5, 28) -> (-91.5, 28)
  line L2 (-91.5, 28) -> (-91.5, -2)
  line L3 (-91.5, -2) -> (-83.5, -2)
  line L4 (-91.5, 28) -> (91.5, 28)
  line L5 (91.5, 28) -> (91.5, -2)
  line L6 (91.5, -2) -> (-91.5, -2)
  line L7 (-91.5, -2) -> (-91.5, 28)
  constraint horizontal L4
  constraint vertical L5
  constraint horizontal L6
  constraint vertical L7
  constraint coincident L1.end L2.start
extrude "Extrude36" add sketch "Sketch30" along normal blind 7 bodies 1
sketch "Sketch31" plane through (0, -87, 0) normal (0, -1, 0) x (1, 0, 0)
  line L0 (-91.5, -2) -> (91.5, -2)
  line L1 (91.5, -2) -> (91.5, 28)
  line L2 (91.5, 28) -> (-91.5, 28)
  line L3 (-91.5, 28) -> (-91.5, -2)
  circle A0 centre (0, 12.5) radius 8
  dimension "d193" = 16
  measures "d193" diameter of A0
extrude "Extrude37" cut sketch "Sketch31" against normal blind 7 contours A0 bodies 1
sketch "Sketch32" plane through (0, -87, 0) normal (0, -1, 0) x (1, 0, 0)
  circle A0 centre (0, 12.5) radius 8
  line L0 (-91.5, -2) -> (91.5, -2)
  line L1 (91.5, -2) -> (91.5, 28)
  line L2 (91.5, 28) -> (-91.5, 28)
  line L3 (-91.5, 28) -> (-91.5, -2)
  circle A1 centre (-40, 12.5) radius 4.5
  circle A2 centre (40, 12.5) radius 4.5
  line L4 (40, 12.5) -> (0, 12.5)
  line L5 (0, 12.5) -> (-40, 12.5)
  dimension "d206" = 9
  dimension "d207" = 9
  dimension "d214" = 40
  dimension "d215" = 40
  constraint coincident A2.centre L4.start
  constraint parallel L2 L4
  constraint parallel L4 L5
  measures "d206" diameter of A1
  measures "d207" diameter of A2
  measures "d214" distance of A2.centre A0.centre
  measures "d215" distance of A0.centre A1.centre
extrude "Extrude38" cut sketch "Sketch32" against normal blind 182 contours A1 | A2 bodies 1
sketch "Sketch35" plane through (0, 0, -2) normal (0, 0, -1) x (1, 0, 0)
  line L0 (-91.5, 87) -> (-91.5, -95)
  line L1 (-91.5, -95) -> (91.5, -95)
  line L2 (91.5, -95) -> (91.5, 87)
  line L3 (91.5, 87) -> (-91.5, 87)
  line L4 (-83.5, 80) -> (83.5, 80)
  line L5 (83.5, 80) -> (83.5, -60)
  line L6 (83.5, -60) -> (65.5, -60)
  line L7 (65.5, -60) -> (65.5, -88)
  line L8 (65.5, -88) -> (-65.5, -88)
  line L9 (-65.5, -88) -> (-65.5, -60)
  line L10 (-65.5, -60) -> (-83.5, -60)
  line L11 (-83.5, -60) -> (-83.5, 80)
  line L12 (-91.5, 87) -> (91.5, 87)
  line L13 (91.5, 87) -> (91.5, -95)
  line L14 (91.5, -95) -> (-91.5, -95)
  line L15 (-91.5, -95) -> (-91.5, 87)
  line L16 (-49.9161, -98) -> (-91.5, -98)
  line L17 (-91.5, -98) -> (-91.5, -95)
  line L18 (-91.5, -95) -> (-49.9161, -95)
  line L19 (-49.9161, -95) -> (-49.9161, -98)
  constraint horizontal L12
  constraint vertical L13
  constraint horizontal L14
  constraint vertical L15
  constraint coincident L1.end L2.start
  constraint coincident L0.start L3.end
  constraint horizontal L16
  constraint vertical L17
  constraint horizontal L18
  constraint vertical L19
  constraint coincident L0.end L1.start
extrude "Extrude41" add sketch "Sketch35" along normal blind 6.65 contours L0 L1 L2 L3 L12 L13 L14 L15 L18 | L4 L5 L6 L7 L8 L9 L10 L11 bodies 1
sketch "Sketch36" plane through (0, 0, -2) normal (0, 0, 1) x (-1, 0, 0)
  line L0 (65.5, -60) -> (83.5, -60)
  line L1 (83.5, -60) -> (83.5, 80)
  line L2 (83.5, 80) -> (-83.5, 80)
  line L3 (-83.5, 80) -> (-83.5, -60)
  line L4 (-83.5, -60) -> (-65.5, -60)
  line L5 (-65.5, -60) -> (-65.5, -88)
  line L6 (-65.5, -88) -> (65.5, -88)
  line L7 (65.5, -88) -> (65.5, -60)
sketch "Sketch37" plane through (0, 0, -2) normal (0, 0, 1) x (-1, 0, 0)
  line L0 (65.5, -60) -> (83.5, -60)
  line L1 (83.5, -60) -> (83.5, 80)
  line L2 (83.5, 80) -> (-83.5, 80)
  line L3 (-83.5, 80) -> (-83.5, -60)
  line L4 (-83.5, -60) -> (-65.5, -60)
  line L5 (-65.5, -60) -> (-65.5, -88)
  line L6 (-65.5, -88) -> (65.5, -88)
  line L7 (65.5, -88) -> (65.5, -60)
  line L8 (-83.5, 80) -> (-59.3, 80)
  line L9 (-59.3, 80) -> (-59.3, -88)
  line L10 (-59.3, -88) -> (-83.5, -88)
  line L11 (-83.5, -88) -> (-83.5, 80)
  line L12 (83.5, 80) -> (59.3, 80)
  line L13 (59.3, 80) -> (59.3, -88)
  line L14 (59.3, -88) -> (83.5, -88)
  line L15 (83.5, -88) -> (83.5, 80)
  dimension "d264" = 24.2
  dimension "d265" = 24.2
  dimension "d266" = 168
  dimension "d267" = 168
  constraint horizontal L8
  constraint vertical L9
  constraint horizontal L10
  constraint vertical L11
  constraint coincident L6 L9.end
  constraint coincident L2.end L3.start
  constraint horizontal L12
  constraint vertical L13
  constraint horizontal L14
  constraint vertical L15
  constraint coincident L1.end L2.start
  measures "d264" distance of L2.end L8.end
  measures "d265" distance of L1.end L12.end
  measures "d266" distance of L8.end L9.end
  measures "d267" distance of L12.end L13.end
extrude "Extrude43" cut sketch "Sketch37" against normal blind 6.65 contours L2 L6 L9 L13 bodies 1
chamfer "Chamfer2" distance 3 angle 45 2 edges at (-59.3, 4, -2) (59.3, 4, -2) on bodies 1
sketch "Sketch39" plane through (0, 95, 0) normal (0, 1, 0) x (-1, 0, 0)
  circle A0 centre (-31.5, 2.5) radius 1.4
  circle A1 centre (31.5, 12.5) radius 1.4
  circle A2 centre (0, 22.5) radius 1.4
  circle A3 centre (-31.5, 12.5) radius 1.4
  circle A4 centre (0, 2.5) radius 1.4
  circle A5 centre (31.5, 22.5) radius 1.4
  circle A6 centre (31.5, 2.5) radius 1.4
  circle A7 centre (-31.5, 22.5) radius 1.4
  circle A8 centre (0, 12.5) radius 4.5
  circle A9 centre (-40, 12.5) radius 4.5
  circle A10 centre (40, 12.5) radius 4.5
  line L0 (-91.5, 28) -> (-91.5, -8.65)
  line L1 (-91.5, -8.65) -> (91.5, -8.65)
  line L2 (91.5, -8.65) -> (91.5, 28)
  line L3 (91.5, 28) -> (-91.5, 28)
  line L4 (-21.15, 33.65) -> (21.15, 33.65)
  line L5 (21.15, 33.65) -> (21.15, -8.65)
  line L6 (21.15, -8.65) -> (-21.15, -8.65)
  line L7 (-21.15, -8.65) -> (-21.15, 33.65)
  circle A11 centre (15.5, 28) radius 1.6
  circle A12 centre (-15.5, 28) radius 1.6
  circle A13 centre (15.5, -3) radius 1.6
  circle A14 centre (-15.5, -3) radius 1.6
  circle A15 centre (-40, 12.5) radius 4.5
  circle A16 centre (40, 12.5) radius 4.5
  circle A17 centre (0, 12.5) radius 8
  line L8 (83.5, -2) -> (83.5, 28)
  line L9 (83.5, 28) -> (-83.5, 28)
  line L10 (-83.5, 28) -> (-83.5, -2)
  line L11 (-83.5, -2) -> (-62.3, -2)
  line L12 (-62.3, -2) -> (-59.3, -5)
  line L13 (-59.3, -5) -> (-59.3, -8.65)
  line L14 (-59.3, -8.65) -> (59.3, -8.65)
  line L15 (59.3, -8.65) -> (59.3, -5)
  line L16 (59.3, -5) -> (62.3, -2)
  line L17 (62.3, -2) -> (83.5, -2)
  circle A18 centre (-40, 12.5) radius 4.5
  circle A19 centre (40, 12.5) radius 4.5
  line L18 (-91.5, 28) -> (-91.5, -8.65)
  line L19 (-91.5, -8.65) -> (91.5, -8.65)
  line L20 (91.5, -8.65) -> (91.5, 28)
  line L21 (91.5, 28) -> (-91.5, 28)
  point P0 (0, 12.5)
  dimension "d287" = 42.3
  dimension "d288" = 3.2
  dimension "d289" = 3.2
  dimension "d290" = 3.2
  dimension "d291" = 3.2
  constraint horizontal L4
  constraint perpendicular L4 L5
  constraint parallel L4 L6
  constraint parallel L5 L7
  constraint coincident P0 A8.centre
  constraint coincident L3 A11.centre
  constraint coincident L3 A12.centre
  measures "d287" distance of L5.end L6.end
  measures "d288" diameter of A11
  measures "d289" diameter of A12
  measures "d290" diameter of A13
  measures "d291" diameter of A14
extrude "Extrude45" add sketch "Sketch39" against normal blind 7 contours L3 L4 L5 L7 A11 A12 L9 L21 bodies 1
extrude "Extrude46" cut sketch "Sketch39" against normal blind 7 contours L3 A12 L9 L21 | L3 A11 L9 L21 | A13 | A14 picked at (-15.6948, 27.5035) picked at (15.3052, 27.3446) bodies 1
extrude "Extrude48" cut 1 faces at (-83.5, 13.3333, 8) along direction (1, 0, 0) blind -30 and the other way blind -220 on bodies 1 bodies 1
sketch "Sketch41" plane through (0, 95, 0) normal (0, -1, 0) x (1, 0, 0)
  circle A0 centre (40, 12.5) radius 4.5
  circle A1 centre (-40, 12.5) radius 4.5
  line L0 (21.15, 28) -> (21.15, 33.65)
  line L1 (21.15, 33.65) -> (-21.15, 33.65)
  line L2 (-21.15, 33.65) -> (-21.15, 28)
  line L3 (-21.15, 28) -> (-65.5, 28)
  line L4 (-59.3, -8.65) -> (59.3, -8.65)
  line L5 (65.5, 28) -> (21.15, 28)
  line L6 (-21.15, 33.65) -> (21.15, 33.65)
  line L7 (21.15, 33.65) -> (21.15, -8.65)
  line L8 (21.15, -8.65) -> (-21.15, -8.65)
  line L9 (-21.15, -8.65) -> (-21.15, 33.65)
  line L10 (-21.15, 33.65) -> (21.15, -8.65) construction
  line L11 (21.15, 33.65) -> (-21.15, -8.65) construction
  line L12 (-12.5, 25) -> (12.5, 25)
  line L13 (12.5, 25) -> (12.5, 0)
  line L14 (12.5, 0) -> (-12.5, 0)
  line L15 (-12.5, 0) -> (-12.5, 25)
  line L16 (-12.5, 25) -> (12.5, 0) construction
  line L17 (12.5, 25) -> (-12.5, 0) construction
  circle A2 centre (0, 12.5) radius 4.5
  line L18 (-65.5, 28) -> (-65.5, -2)
  line L19 (-65.5, -2) -> (-62.3, -2)
  line L20 (-62.3, -2) -> (-59.3, -5)
  line L21 (-59.3, -5) -> (-59.3, -8.65)
  line L22 (59.3, -8.65) -> (59.3, -5)
  line L23 (59.3, -5) -> (62.3, -2)
  line L24 (62.3, -2) -> (65.5, -2)
  line L25 (65.5, -2) -> (65.5, 28)
  circle A3 centre (15.5, 28) radius 1.6
  circle A4 centre (-15.5, 28) radius 1.6
  circle A5 centre (15.5, -3) radius 1.6
  circle A6 centre (-15.5, -3) radius 1.6
  line L26 (21.15, 28) -> (91.5, 28)
  line L27 (91.5, 28) -> (91.5, -8.65)
  line L28 (91.5, -8.65) -> (-91.5, -8.65)
  line L29 (-91.5, -8.65) -> (-91.5, 28)
  line L30 (-91.5, 28) -> (-21.15, 28)
  line L31 (-21.15, 28) -> (-21.15, 33.65)
  line L32 (-21.15, 33.65) -> (21.15, 33.65)
  line L33 (21.15, 33.65) -> (21.15, 28)
  circle A7 centre (40, 12.5) radius 4.5
  circle A8 centre (-40, 12.5) radius 4.5
  point P0 (0, 12.5)
  point P1 (0, 12.5)
  dimension "d308" = 25
  dimension "d309" = 25
  constraint horizontal L6
  constraint perpendicular L6 L7
  constraint parallel L6 L8
  constraint parallel L7 L9
  constraint coincident L10 P1
  constraint coincident L11 P1
  constraint coincident L1.end L2.start
  constraint horizontal L12
  constraint perpendicular L12 L13
  constraint parallel L12 L14
  constraint parallel L13 L15
  constraint coincident L16 P1
  constraint coincident L17 P1
  measures "d308" distance of L13.end L14.end
  measures "d309" distance of L12.end L13.end
extrude "Extrude49" add sketch "Sketch41" against normal blind 17.7 contours L0 L1 L2 L4 L6 L7 L8 L9 L28 L31 L32 L33 bodies 1
sketch "Sketch42" plane through (0, -80, 0) normal (0, 1, 0) x (-1, 0, 0)
  line L0 (91.5, 28) -> (-91.5, 28)
  line L1 (-91.5, 28) -> (-91.5, -2)
  line L2 (-91.5, -2) -> (-62.3, -2)
  line L3 (-62.3, -2) -> (-59.3, -5)
  line L4 (-59.3, -5) -> (-59.3, -8.65)
  line L5 (-59.3, -8.65) -> (59.3, -8.65)
  line L6 (59.3, -8.65) -> (59.3, -5)
  line L7 (59.3, -5) -> (62.3, -2)
  line L8 (62.3, -2) -> (91.5, -2)
  line L9 (91.5, -2) -> (91.5, 28)
  circle A0 centre (0, 12.5) radius 8
  circle A1 centre (40, 12.5) radius 4.5
  circle A2 centre (-40, 12.5) radius 4.5
  line L10 (-91.5, 28) -> (-51.5, 28)
  line L11 (-51.5, 28) -> (-51.5, -2)
  line L12 (-51.5, -2) -> (-91.5, -2)
  line L13 (-91.5, -2) -> (-91.5, 28)
  line L14 (91.5, 28) -> (51.5, 28)
  line L15 (51.5, 28) -> (51.5, -2)
  line L16 (51.5, -2) -> (91.5, -2)
  line L17 (91.5, -2) -> (91.5, 28)
  dimension "d312" = 40
  dimension "d313" = 40
  constraint horizontal L10
  constraint vertical L11
  constraint horizontal L12
  constraint vertical L13
  constraint coincident L0.end L1.start
  constraint horizontal L14
  constraint vertical L15
  constraint horizontal L16
  constraint vertical L17
  constraint coincident L0.start L9.end
  measures "d312" distance of L0.end L10.end
  measures "d313" distance of L0.start L14.end
extrude "Extrude50" cut sketch "Sketch42" against normal blind 35 contours L0 L8 L9 L14 L15 L16 L17 | L0 L1 L2 L10 L11 L12 L13 bodies 1
extrude "Extrude51" cut 2 faces at (91.5, 22.6667, -6.4333) (91.5, 87.9846, 12.8333) along direction (-1, 0, 0) blind 15 on bodies 1 bodies 1